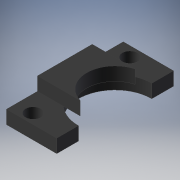
# Autodesk Inventor part: UCover_PWR
Saved by Autodesk Inventor 2019.4 (Build 234330000, 330)
## iProperties
Created: 2020-06-11
Part Number: UCover_PWR
Material: Generic
Document SubType Name: Modeling
Designer: ions
Density: 1 g/cm^3
Appearance: Default
Mass: 0.1443 g
Surface Area: 2.83872 cm^2
Volume: 0.1443 cm^3
Author: ions
Autodesk Inventor part; units mm, degrees
ref_plane "YZ Plane" through (0, 0, 0) normal (1, 0, 0) x (0, 1, 0)
ref_plane "XZ Plane" through (0, 0, 0) normal (0, 1, 0) x (-1, 0, 0)
ref_plane "XY Plane" through (0, 0, 0) normal (0, 0, 1) x (1, 0, 0)
sketch "Sketch1" plane through (0, 0, 0) normal (0, 1, 0) x (-1, 0, 0)
  line L0 (-0.3136, 9.3425) -> (-7.8416, 9.3425)
  line L1 (-7.8416, -8.1575) -> (-0.3136, -8.1575)
  line L2 (-0.3136, -8.1575) -> (-0.3136, 9.3425)
  circle A0 centre (-2.8136, 7.8425) radius 1.15
  circle A1 centre (-2.8136, -6.6575) radius 1.15
  arc A2 (-7.8416, -3.6575) -> (-7.8416, 4.8425) centre (-7.8416, 0.5925) ccw
  line L3 (-7.8416, 9.3425) -> (-7.8416, 4.8425)
  line L4 (-7.8416, -3.6575) -> (-7.8416, -8.1575)
  point P0 (0, 0)
  point P1 (0, 0)
  dimension "d0" = 17.5
  dimension "d1" = 2.5
  dimension "d2" = 2.5
  dimension "d3" = 1.5
  dimension "d4" = 1.5
  dimension "d5" = 2.3
  dimension "d6" = 2.3
  dimension "d7" = 8.5
  dimension "d8" = 7.528
  dimension "d9" = 8.75
  constraints: 10 end point, 3 centre point, 3 parallel, 2 perpendicular, 2 point on circle, 1 horizontal
  measures "d0" distance between parallel lines of L1 L0
  measures "d1" distance from line of A0.centre L2
  measures "d2" distance from line of A1.centre L2
  measures "d3" distance from line of L0 A0.centre
  measures "d4" distance from line of L1 A1.centre
  measures "d5" diameter of A0
  measures "d6" diameter of A1
  measures "d7" diameter of A2
  measures "d8" distance between parallel lines of L3 L2
  measures "d9" distance from line of A2.centre L0
extrude "Extrusion1" add sketch "Sketch1" along normal blind 4
sketch "Sketch3" plane through (0, 0, 0) normal (0, -1, 0) x (1, 0, 0)
  circle A0 centre (7.8416, 0.5925) radius 5.5
  line L0 (7.8416, 9.3425) -> (7.8416, 4.8425) projected
  line L1 (7.8416, -8.1575) -> (0.3136, -8.1575) projected
  point P0 (0, 0)
  dimension "d12" = 11
  dimension "d13" = 0
  dimension "d14" = 8.75
  constraints: 1 centre point
  measures "d12" diameter of A0
  measures "d13" distance from line of L0 A0.centre
  measures "d14" distance from line of L1 A0.centre
extrude "Extrusion2" cut sketch "Sketch3" against normal blind 2
sketch "Sketch4" plane through (0, 4, 0) normal (0, 1, 0) x (1, 0, 0)
  line L0 (7.8416, -9.3425) -> (0.3136, -9.3425)
  line L1 (0.3136, -9.3425) -> (0.3136, -4.6925)
  line L2 (0.3136, -4.6925) -> (7.8416, -4.6925)
  line L3 (7.8416, -4.6925) -> (7.8416, -9.3425)
  line L4 (7.8416, 3.6575) -> (7.8416, 8.1575) projected
  line L5 (0.3136, 8.1575) -> (0.3136, -9.3425) projected
  line L6 (7.8416, 8.1575) -> (0.3136, 8.1575)
  line L7 (0.3136, 8.1575) -> (0.3136, 3.5075)
  line L8 (0.3136, 3.5075) -> (7.8416, 3.5075)
  line L9 (7.8416, 3.5075) -> (7.8416, 8.1575)
  point P0 (0, 0)
  dimension "d17" = 4.65
  dimension "d18" = 4.65
  dimension "d23" = 0
  constraints: 16 end point, 4 parallel, 2 horizontal, 2 perpendicular, 1 point on line
  measures "d17" distance between parallel lines of L2 L0
  measures "d18" distance between parallel lines of L6 L8
  measures "d23" distance between parallel lines of L5 L1
extrude "Extrusion3" cut sketch "Sketch4" against normal blind 2 contours L0 L1 L2 L3
extrude "Extrusion4" cut sketch "Sketch4" against normal blind 2 contours L5 L6 L4 L9 L8
body "Solid1"
